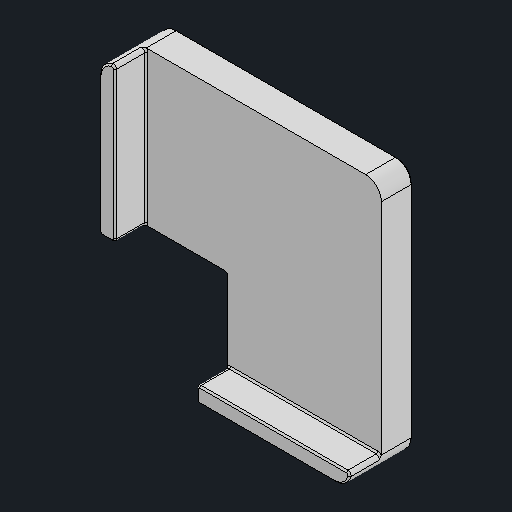
# Autodesk Inventor part: corner-cutting-jig-31mm
Saved by Autodesk Inventor 2026 (Build 300175050, 175E)
## iProperties
Created: 2026-05-15
Part Number: corner-cutting-jig-31mm
Material: Generic
Document SubType Name: Modeling
Designer: kuzmin
Density: 1 g/cm^3
Appearance: Default
Author: kuzmin
Autodesk Inventor part; units mm, degrees
ref_plane "YZ Plane" through (0, 0, 0) normal (1, 0, 0) x (0, 1, 0)
ref_plane "XZ Plane" through (0, 0, 0) normal (0, 1, 0) x (-1, 0, 0)
ref_plane "XY Plane" through (0, 0, 0) normal (0, 0, 1) x (1, 0, 0)
sketch "Sketch1" plane through (0, 0, 0) normal (0, 0, 1) x (1, 0, 0)
  line L0 (-40, 40) -> (40, 40)
  line L1 (40, 40) -> (40, -40)
  line L2 (40, -40) -> (-40, -40)
  line L3 (-40, -40) -> (-40, 40)
  point P0 (0, 0)
  point P1 (0, 40)
  point P2 (40, 0)
  dimension "d0" = 80
  constraints: 8 end point, 2 midpoint, 2 parallel, 2 perpendicular, 1 horizontal, 1 horizontal alignment, 1 vertical alignment
  measures "d0" distance of L0.start L0.end
extrude "Extrusion1" add sketch "Sketch1" along normal blind 20
sketch "Sketch3" plane through (0, 0, 20) normal (0, 0, 1) x (1, 0, 0)
  line L0 (40, -40) -> (40, 40) projected
  line L1 (-35, -35) -> (40, -35)
  line L2 (40, -35) -> (40, 40)
  line L3 (40, 40) -> (-35, 40)
  line L4 (-35, 40) -> (-35, -35)
  line L5 (-40, 40) -> (-40, -40) projected
  line L6 (-40, -40) -> (40, -40) projected
  line L7 (-35, 40) -> (-40, 40)
  line L8 (40, -35) -> (40, -40)
  point P0 (0, 0)
  dimension "d9" = 5
  dimension "d10" = 5
  constraints: 12 end point, 2 horizontal, 2 parallel, 2 perpendicular
  measures "d9" distance between parallel lines of L4 L5
  measures "d10" distance between parallel lines of L6 L1
extrude "Extrusion3" cut sketch "Sketch3" against normal blind 10 contours L1 L4 L3 L0
sketch "Sketch2" plane through (0, 0, 20) normal (0, 0, 1) x (1, 0, 0)
  line L0 (-50, -9) -> (-9, -9)
  line L1 (-9, -9) -> (-9, -50)
  line L2 (-9, -50) -> (-50, -50)
  line L3 (-50, -50) -> (-50, -9)
  line L4 (-40, 40) -> (-40, -40) projected
  line L5 (-40, -40) -> (40, -40) projected
  point P0 (0, 0)
  point P1 (-9, -40)
  point P2 (-40, -9)
  dimension "d3" = 31
  dimension "d4" = 31
  dimension "d5" = 10
  dimension "d6" = 10
  constraints: 8 end point, 2 parallel, 1 horizontal, 1 perpendicular
  measures "d3" distance between parallel lines of L1 L4
  measures "d4" distance between parallel lines of L5 L0
  measures "d5" distance between parallel lines of L2 L5
  measures "d6" distance between parallel lines of L3 L4
extrude "Extrusion2" cut sketch "Sketch2" against normal through all contours L0 L1 L5 L4
fillet "Fillet1" radius 5 3 edges at (40, 40, 5) (-40, 40, 10) (40, -40, 10)
fillet "Fillet2" radius 1 7 edges at (-35, 40, 15) (40, -35, 15) (-9, -35, 15) (-35, -9, 15) (-40, -9, 10) (-9, -40, 10) (-9, -9, 5)
chamfer "Chamfer1" distance 0.5 angle 45 32 edges at (40, 0, 0) (38.5355, 38.5355, 0) (0, 40, 0) (-38.5355, 38.5355, 0) (-40, 13.5, 0) (-39.7071, -8.7071, 0) (-24.5, -9, 0) (-9.2929, -9.2929, 0) (-9, -24.5, 0) (-8.7071, -39.7071, 0) (13.5, -40, 0) (38.5355, -38.5355, 0) (-35, 15.4365, 10) (-35.3876, 39.6636, 10) (-35.2929, -8.7071, 10) (15.4365, -35, 10) (-8.7071, -35.2929, 10) (39.6636, -35.3876, 10) (-35, 15.4365, 20) (-35.3876, 39.6636, 20) (-38.9528, 38.0619, 20) (-40, 13.5, 20) (-39.7071, -8.7071, 20) (-37.5, -9, 20) (-35.2929, -8.7071, 20) (15.4365, -35, 20) (-8.7071, -35.2929, 20) (-9, -37.5, 20) (-8.7071, -39.7071, 20) (13.5, -40, 20) (38.0619, -38.9528, 20) (39.6636, -35.3876, 20)
body "Solid1"
